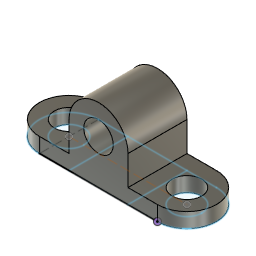
A4 piece v2 (Autodesk Fusion 360 design; units mm, degrees)
Autodesk Fusion 360 part; units mm, degrees
sketch "top view" plane through (0, 0, 0) normal (0, 0, 1) x (1, 0, 0)
  line L0 (0, 0) -> (-80, 0)
  line L1 (-80, 0) -> (-80, 40) construction
  line L2 (-80, 40) -> (0, 40)
  arc A0 (-80, 40) -> (-80, 0) centre (-80, 20) ccw
  arc A1 (0, 0) -> (0, 40) centre (0, 20) ccw
  line L3 (-80, 20) -> (0, 20) construction
  line L4 (-60, 40) -> (-60, 0)
  line L5 (-20, 40) -> (-20, 0)
  circle A2 centre (-80, 20) radius 10
  circle A3 centre (0, 20) radius 10
  dimension "d1" = 40
  dimension "d2" = 80
  constraint horizontal L0
  constraint vertical L1
  constraint horizontal L2
  constraint coincident L0.start A1.start
  constraint midpoint L1 A0.centre
  constraint coincident A0.centre L3.start
  constraint coincident A1.centre L3.end
  constraint perpendicular L1 L3
  constraint coincident L2 L4.start
  constraint coincident L0 L4.end
  constraint perpendicular L0 L4
  constraint coincident L2 L5.start
  constraint coincident L0 L5.end
  constraint perpendicular L0 L5
  constraint concentric A0 A2
  constraint concentric A1 A3
  measures "d1" distance of L0.start L2.end
  measures "d2" distance of L0.start L0.end
extrude "Extrude1" add sketch "top view" along normal blind 10
extrude "Extrude2" add sketch "top view" along normal blind 50 contours L0 L2 L4 L5
fillet "Fillet1" radius 20 2 edges at (-20, 20, 50) (-60, 20, 50)
hole "Hole2" at (-40, 40, 30) direction (0, -1, 0) diameter 20 end through all
equation "d2 = 20 mm + 40 mm + 20 mm"
named bodies: "A4"
